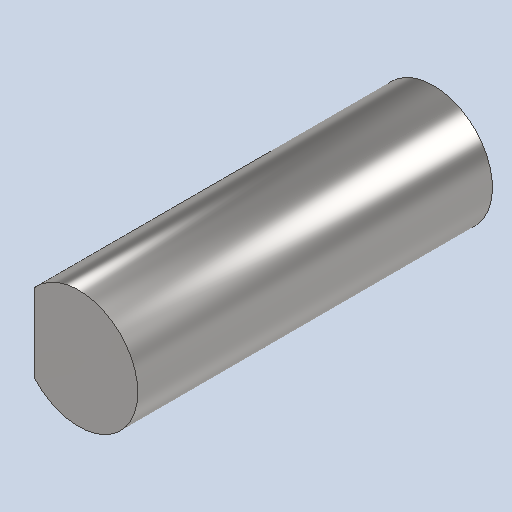
# Autodesk Inventor part: 軸
Saved by Autodesk Inventor 2024 (Build 280153000, 153)
## iProperties
Created: 2024-03-31
Part Number: 軸
Material: 不鏽鋼
Document SubType Name: Modeling
Designer: USER
Density: 8 g/cm^3
Appearance: 半拋光
Author: USER
Autodesk Inventor part; units mm, degrees
ref_plane "YZ Plane" through (0, 0, 0) normal (1, 0, 0) x (0, 1, 0)
ref_plane "XZ Plane" through (0, 0, 0) normal (0, 1, 0) x (-1, 0, 0)
ref_plane "XY Plane" through (0, 0, 0) normal (0, 0, 1) x (1, 0, 0)
sketch "草圖1" plane through (0, 0, 0) normal (1, 0, 0) x (0, 1, 0)
  line L0 (2, 0) -> (-2, 0)
  line L1 (-2, 0) -> (-2, -12)
  line L2 (-2, -12) -> (2, -12)
  line L3 (2, -12) -> (2, 0)
  line L4 (0, 0) -> (0, -12)
  dimension "d0" = 12
  dimension "d1" = 4
  constraints: 10 end point, 2 midpoint, 2 parallel, 1 coincident, 1 horizontal, 1 perpendicular
  measures "d0" distance of L2.end L0.start
  measures "d1" distance of L1.end L2.end
revolve "迴轉1" add sketch "草圖1" angle 360 about axis through (0, 0, 0) along (0, 0, -1) contours L3 L2 L4 L0
sketch "草圖2" plane through (0, 0, 0) normal (0, 0, 1) x (1, 0, 0)
  circle A0 centre (0, 0) radius 2
  line L0 (-1.5, 1.3229) -> (-1.5, -1.3229)
  dimension "d3" = 4
  dimension "d4" = 1.5
  constraints: 2 end point, 2 point on circle, 1 centre point, 1 coincident, 1 vertical
  measures "d3" diameter of A0
  measures "d4" distance from line of L0 point (0, 0)
extrude "擠出1" cut sketch "草圖2" against normal blind 8 contours L0 A0 picked at (-1.5908, -0.3089)
